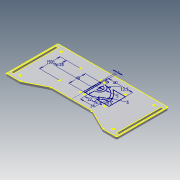
# Autodesk Inventor part: FrontPanel
Saved by Autodesk Inventor 2014 (Build 180170000, 170)
## iProperties
Created: 2015-01-19
Part Number: FrontPanel
Material: Generic
Document SubType Name: Modeling
Designer: Peele
Density: 1 g/cm^3
Appearance: White
Author: Peele
Autodesk Inventor part; units mm, degrees
ref_plane "YZ Plane" through (0, 0, 0) normal (1, 0, 0) x (0, 1, 0)
ref_plane "XZ Plane" through (0, 0, 0) normal (0, 1, 0) x (-1, 0, 0)
ref_plane "XY Plane" through (0, 0, 0) normal (0, 0, 1) x (1, 0, 0)
sketch "Sketch1" plane through (0, 0, 0) normal (0, 0, 1) x (1, 0, 0)
  line L0 (0, 0) -> (0, 125)
  line L1 (0, 125) -> (268, 125)
  line L2 (268, 125) -> (268, 0)
  line L3 (268, 0) -> (0, 0)
  point P0 (134, 125)
  dimension "d1" = 125
  dimension "d2" = 268
  constraints: 8 end point, 2 horizontal, 2 vertical, 1 midpoint
  measures "d1" distance of L1.end L2.end
  measures "d2" distance of L2.end L0.start
extrude "Extrusion1" add sketch "Sketch1" along normal blind 6
sketch "Sketch2" plane through (0, 0, 6) normal (0, 0, 1) x (1, 0, 0)
  line L0 (0, 0) -> (268, 0) projected
  line L1 (268, 0) -> (268, 125) projected
  line L2 (34, 0) -> (84, 25)
  line L3 (84, 25) -> (184, 25)
  line L4 (184, 25) -> (234, 0)
  line L5 (234, 0) -> (34, 0)
  line L6 (0, 125) -> (0, 0) projected
  dimension "d6" = 25
  dimension "d7" = 34
  dimension "d9" = 50
  dimension "d47" = 34
  constraints: 8 end point, 2 point on line, 1 collinear, 1 equal length, 1 parallel
  measures "d6" distance between parallel lines of L0 L3
  measures "d7" distance from line of L4.end L1
  measures "d9" horizontal distance of L2.end L2.start
  measures "d47" distance from line of L6 L2.start
extrude "Extrusion2" cut sketch "Sketch2" against normal through all
sketch "Sketch7" plane through (0, 0, 6) normal (0, 0, 1) x (1, 0, 0)
  line L0 (268, 0) -> (268, 125) projected
  line L1 (268, 125) -> (0, 125) projected
  line L2 (0, 125) -> (0, 0) projected
  line L3 (0, 0) -> (34, 0) projected
  circle A0 centre (246.5, 12.5) radius 2.7
  circle A1 centre (246.5, 112.5) radius 2.7
  circle A2 centre (21.5, 12.5) radius 2.7
  circle A3 centre (21.5, 112.5) radius 2.7
  line L4 (2.875, 8.1) -> (9.125, 8.1)
  line L5 (9.125, 8.1) -> (9.125, 117)
  line L6 (9.125, 117) -> (2.875, 117)
  line L7 (2.875, 117) -> (2.875, 8.1)
  line L8 (2.875, 8.1) -> (9.125, 117) construction
  line L9 (9.125, 8.1) -> (2.875, 117) construction
  line L10 (258.875, 8.1) -> (265.125, 8.1)
  line L11 (265.125, 8.1) -> (265.125, 117)
  line L12 (265.125, 117) -> (258.875, 117)
  line L13 (258.875, 117) -> (258.875, 8.1)
  line L14 (258.875, 8.1) -> (265.125, 117) construction
  line L15 (265.125, 8.1) -> (258.875, 117) construction
  point P0 (6, 62.55)
  point P1 (262, 62.55)
  point P2 (6, 62.55)
  point P3 (262, 62.55)
  dimension "d48" = 21.5
  dimension "d49" = 21.5
  dimension "d50" = 12.5
  dimension "d51" = 12.5
  dimension "d56" = 2.875
  dimension "d57" = 6.25
  dimension "d58" = 2.875
  dimension "d60" = 8
  dimension "d61" = 5.4
  dimension "d62" = 108.9
  dimension "d66" = 8.1
  constraints: 24 end point, 6 midpoint, 4 centre point, 4 parallel, 3 equal radius, 3 horizontal alignment, 2 equal length, 2 horizontal, 2 perpendicular, 2 vertical alignment
  measures "d48" distance from line of A3.centre L2
  measures "d49" distance from line of A1.centre L0
  measures "d50" distance from line of A3.centre L1
  measures "d51" distance from line of A2.centre L3
  measures "d56" distance between parallel lines of L2 L7
  measures "d57" distance of L5.end L6.end
  measures "d58" distance between parallel lines of L11 L0
  measures "d60" distance between parallel lines of L1 L6
  measures "d61" diameter of A3
  measures "d62" distance of L4.end L5.end
  measures "d66" distance between parallel lines of L4 L3
extrude "Extrusion5" cut sketch "Sketch7" against normal through all
fillet "Fillet1" radius 2 8 edges at (268, 125, 3) (268, 0, 3) (234, 0, 3) (184, 25, 3) (84, 25, 3) (34, 0, 3) (0, 0, 3) (0, 125, 3)
sketch "Sketch8" plane through (0, 0, 6) normal (0, 0, 1) x (1, 0, 0)
  line L0 (9.125, 8.1) -> (2.875, 8.1) projected
  line L1 (84.4721, 25) -> (183.5279, 25) projected
  line L2 (266, 125) -> (2, 125) projected
  line L3 (79, 50) -> (129, 50) construction
  line L4 (129, 50) -> (129, 100) construction
  line L5 (129, 100) -> (79, 100) construction
  line L6 (79, 100) -> (79, 50) construction
  line L7 (79, 50) -> (129, 100) construction
  line L8 (129, 50) -> (79, 100) construction
  line L9 (139, 50) -> (189, 50) construction
  line L10 (189, 50) -> (189, 100) construction
  line L11 (189, 100) -> (139, 100) construction
  line L12 (139, 100) -> (139, 50) construction
  line L13 (139, 50) -> (189, 100) construction
  line L14 (189, 50) -> (139, 100) construction
  line L15 (104, 75) -> (164, 75) construction
  line L16 (134, 75) -> (134, 25) construction
  circle A0 centre (79, 100) radius 2.15
  circle A1 centre (129, 100) radius 2.15
  circle A2 centre (139, 100) radius 2.15
  circle A3 centre (189, 100) radius 2.15
  circle A4 centre (189, 50) radius 2.15
  circle A5 centre (139, 50) radius 2.15
  circle A6 centre (129, 50) radius 2.15
  circle A7 centre (79, 50) radius 2.15
  point P0 (0, 0)
  dimension "d67" = 50
  dimension "d68" = 60
  dimension "d69" = 100
  dimension "d70" = 25
  dimension "d71" = 4.3
  constraints: 28 end point, 8 centre point, 8 coincident, 7 equal radius, 6 midpoint, 5 parallel, 3 equal length, 3 perpendicular, 2 horizontal, 1 vertical
  measures "d67" distance of L4.end L5.end
  measures "d68" distance of L15.end L15.start
  measures "d69" distance between parallel lines of L2 L1
  measures "d70" distance between parallel lines of L2 L5
  measures "d71" diameter of A3
extrude "Extrusion6" cut sketch "Sketch8" against normal blind 10
sketch "Sketch9" plane through (0, 0, 6) normal (0, 0, 1) x (1, 0, 0)
  circle A0 centre (129, 50) radius 2.15 projected
  circle A1 centre (189, 50) radius 2.15 projected
  circle A2 centre (139, 100) radius 2.15 projected
  circle A3 centre (79, 100) radius 2.15 projected
  circle A4 centre (129, 100) radius 2.15 projected
  circle A5 centre (189, 100) radius 2.15 projected
  circle A6 centre (139, 50) radius 2.15 projected
  circle A7 centre (79, 50) radius 2.15 projected
  line L0 (9.125, 117) -> (9.125, 8.1) projected
  line L1 (9.125, 8.1) -> (2.875, 8.1) projected
  line L2 (2.875, 8.1) -> (2.875, 117) projected
  line L3 (2.875, 117) -> (9.125, 117) projected
  circle A8 centre (21.5, 12.5) radius 2.7 projected
  circle A9 centre (246.5, 12.5) radius 2.7 projected
  circle A10 centre (246.5, 112.5) radius 2.7 projected
  circle A11 centre (21.5, 112.5) radius 2.7 projected
  line L4 (265.125, 117) -> (265.125, 8.1) projected
  line L5 (265.125, 8.1) -> (258.875, 8.1) projected
  line L6 (258.875, 8.1) -> (258.875, 117) projected
  line L7 (258.875, 117) -> (265.125, 117) projected
  arc A12 (2, 125) -> (0, 123) centre (2, 123) ccw projected
  line L8 (0, 123) -> (0, 2) projected
  arc A13 (0, 2) -> (2, 0) centre (2, 2) ccw projected
  line L9 (2, 0) -> (33.5279, 0) projected
  arc A14 (33.5279, 0) -> (34.4223, 0.2111) centre (33.5279, 2) ccw projected
  line L10 (34.4223, 0.2111) -> (83.5777, 24.7889) projected
  arc A15 (84.4721, 25) -> (83.5777, 24.7889) centre (84.4721, 23) ccw projected
  line L11 (84.4721, 25) -> (183.5279, 25) projected
  arc A16 (184.4223, 24.7889) -> (183.5279, 25) centre (183.5279, 23) ccw projected
  line L12 (184.4223, 24.7889) -> (233.5777, 0.2111) projected
  arc A17 (233.5777, 0.2111) -> (234.4721, 0) centre (234.4721, 2) ccw projected
  line L13 (234.4721, 0) -> (266, 0) projected
  arc A18 (266, 0) -> (268, 2) centre (266, 2) ccw projected
  line L14 (268, 2) -> (268, 123) projected
  arc A19 (268, 123) -> (266, 125) centre (266, 123) ccw projected
  line L15 (266, 125) -> (2, 125) projected
  line L16 (132, 55) -> (136, 55)
  line L17 (136, 55) -> (136, 95)
  line L18 (136, 95) -> (132, 95)
  line L19 (132, 95) -> (132, 55)
  line L20 (132, 55) -> (136, 95) construction
  line L21 (136, 55) -> (132, 95) construction
  line L22 (134, 25) -> (134, 75) construction
  line L23 (144, 90) -> (144, 75)
  arc A20 (144, 75) -> (144, 90) centre (144, 82.5) ccw
  arc A21 (144, 70) -> (144, 95) centre (144, 82.5) ccw
  line L24 (144, 70) -> (144, 55)
  arc A22 (178, 70) -> (144, 95) centre (144, 59.38) ccw
  arc A23 (178, 70) -> (166, 64) centre (181.2699, 48.4602) ccw
  arc A24 (144, 55) -> (166, 64) centre (144, 86.3889) ccw
  line L25 (144, 95) -> (136, 95) construction
  line L26 (136, 55) -> (144, 55) construction
  line L27 (163.5243, 95) -> (194, 95)
  line L28 (194, 95) -> (194, 55)
  line L29 (194, 55) -> (163, 55)
  arc A25 (184.2317, 64.9834) -> (163.5243, 95) centre (144, 59.38) ccw
  arc A26 (162.4089, 55) -> (169.5044, 60.4336) centre (144, 86.3889) ccw
  arc A27 (184.2317, 64.9834) -> (169.5044, 60.4336) centre (181.2699, 48.4602) ccw
  point P0 (0, 0)
  point P1 (140, 55)
  dimension "d74" = 4
  dimension "d75" = 40
  dimension "d76" = 50
  dimension "d77" = 25
  dimension "d78" = 12.5
  dimension "d79" = 5
  dimension "d80" = 8
  dimension "d81" = 22
  dimension "d82" = 15
  dimension "d83" = 34
  dimension "d84" = 9
  dimension "d85" = 5
  dimension "d86" = 5
  dimension "d87" = 60
  constraints: 28 end point, 16 point on circle, 8 centre point, 7 parallel, 5 tangent, 4 collinear, 4 concentric, 4 midpoint, 3 horizontal, 2 perpendicular, 1 point on line, 1 vertical
  measures "d74" distance of L17.end L18.end
  measures "d75" distance of L18.end L16.start
  measures "d76" distance of A7.centre A3.centre
  measures "d77" vertical distance of L22.end A3.centre
  measures "d78" radius of A21
  measures "d79" radial gap between concentric circles of A21 A20
  measures "d80" distance between parallel lines of L17 L23
  measures "d81" distance from line of A23.end L24
  measures "d82" distance from line of A22.start L16
  measures "d83" distance from line of A22.start L24
  measures "d84" distance from line of A23.end L16
  measures "d85" radial gap between concentric circles of A25 A22
  measures "d86" radial gap between concentric circles of A24 A26
  measures "d87" distance from line of L22.end L28
equation "\"d7\" = d47"
equation "\"d49\" = d48"
equation "\"d51\" = d50"
equation "\"d58\" = d56"
equation "\"d70\" = -0.5 * d67 + 0.5 * d69"
equation "\"d77\" = 0.5 * d76"
equation "\"d86\" = d85"
body "Solid1"
